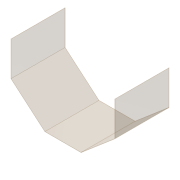
# Autodesk Inventor part: Shroud
Saved by Autodesk Inventor 2012 (Build 160160000, 160)
## iProperties
Created: 2012-02-26
Part Number: Shroud
Material: Polycarbonate, Smoke
Document SubType Name: Modeling
Designer: JesseK
Density: 1.2 g/cm^3
Mass: 1272.09 g
Surface Area: 6766.53 cm^2
Volume: 1060.07 cm^3
Author: JesseK
Autodesk Inventor part; units mm, degrees
ref_plane "YZ Plane" through (0, 0, 0) normal (1, 0, 0) x (0, 1, 0)
ref_plane "XZ Plane" through (0, 0, 0) normal (0, 1, 0) x (-1, 0, 0)
ref_plane "XY Plane" through (0, 0, 0) normal (0, 0, 1) x (1, 0, 0)
sketch "Sketch1" plane through (0, 0, 0) normal (0, 0, 1) x (1, 0, 0)
  line L0 (0, 0) -> (0, -194.0165)
  line L1 (0, -194.0165) -> (191.5029, -357.1875)
  line L2 (191.5029, -357.1875) -> (395.8721, -357.1875)
  line L3 (395.8721, -357.1875) -> (587.375, -194.0165)
  line L4 (587.375, -194.0165) -> (587.375, 0)
  line L5 (0, 0) -> (1.5875, 0)
  line L6 (1.5875, 0) -> (1.5875, -193.2836)
  line L7 (1.5875, -193.2836) -> (192.0875, -355.6)
  line L8 (192.0875, -355.6) -> (395.2875, -355.6)
  line L9 (395.2875, -355.6) -> (585.7875, -193.2836)
  line L10 (585.7875, -193.2836) -> (585.7875, 0)
  line L11 (585.7875, 0) -> (587.375, 0)
  dimension "d0" = 1.5875
  dimension "d1" = 1.5875
  dimension "d2" = 1.5875
  dimension "d3" = 355.6
  dimension "d4" = 584.2
  dimension "d5" = 203.2
  constraints: 24 end point, 5 equal length, 4 horizontal, 4 vertical, 2 parallel, 1 collinear
  measures "d0" distance between parallel lines of L6 L0
  measures "d1" distance between parallel lines of L7 L1
  measures "d2" distance between parallel lines of L2 L8
  measures "d3" distance between parallel lines of L8 L5
  measures "d4" distance between parallel lines of L10 L6
  measures "d5" distance of L7.end L8.end
extrude "Extrusion1" add sketch "Sketch1" along normal blind 304.8
body "Solid1"
